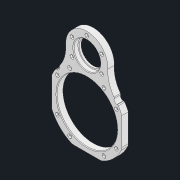
# Autodesk Inventor part: base5
Saved by Autodesk Inventor 2022 (Build 260153000, 153)
## iProperties
Created: 2021-09-16
Part Number: base5
Material: ABS プラスチック
Document SubType Name: Modeling
Designer: Yuta Kage
Density: 1.06 g/cm^3
Appearance: 滑らか - 白
Author: Yuta Kage
Autodesk Inventor part; units mm, degrees
ref_plane "YZ Plane" through (0, 0, 0) normal (1, 0, 0) x (0, 1, 0)
ref_plane "XZ Plane" through (0, 0, 0) normal (0, 1, 0) x (-1, 0, 0)
ref_plane "XY Plane" through (0, 0, 0) normal (0, 0, 1) x (1, 0, 0)
sketch "スケッチ1" plane through (0, 0, 0) normal (0, 0, 1) x (1, 0, 0)
  circle A0 centre (0, 0) radius 47.5 construction
  circle A1 centre (0, 76.8) radius 21 construction
  circle A2 centre (0, 0) radius 59.5
  circle A3 centre (0, 76.8) radius 33
  line L0 (-55.8457, 20.5306) -> (-30.9733, 88.1867)
  line L1 (30.9733, 88.1867) -> (55.8457, 20.5306)
  line L2 (-55, 131.8) -> (55, 131.8)
  line L3 (55, 131.8) -> (55, -55)
  line L4 (55, -55) -> (-55, -55)
  line L5 (-55, -55) -> (-55, 131.8)
  line L6 (-55, 131.8) -> (55, -55) construction
  line L7 (55, 131.8) -> (-55, -55) construction
  line L8 (0, 76.8) -> (-55, 131.8)
  point P0 (0, 38.4)
  point P1 (0, 38.4)
  point P2 (55, 22.8311)
  point P3 (-55, 22.8311)
  point P4 (-55, -22.6991)
  point P5 (-22.6991, -55)
  point P6 (22.6991, -55)
  point P7 (55, -22.6991)
  point P8 (-55, 22.6991)
  point P9 (55, 22.6991)
  point P10 (24.1948, 54.3587)
  point P11 (-24.1948, 54.3587)
  dimension "d0" = 95
  dimension "d1" = 42
  dimension "d2" = 76.8
  dimension "d3" = 12
  dimension "d4" = 12
  dimension "d65" = 110
  dimension "d66" = 38.4
  dimension "d68" = 45
  constraints: 18 end point, 4 centre point, 4 point on circle, 4 tangent, 3 midpoint, 2 parallel, 2 vertical alignment, 1 coincident, 1 horizontal, 1 perpendicular
  measures "d0" diameter of A0
  measures "d1" diameter of A1
  measures "d2" distance of point (0, 0) L8.start
  measures "d3" radial gap between concentric circles of A0 A2
  measures "d4" radial gap between concentric circles of A1 A3
  measures "d65" distance of L3.end L4.end
  measures "d66" distance of point (0, 0) point (0, 38.4)
  measures "d68" angle of L2 L8
extrude "押し出し1" add sketch "スケッチ1" along normal blind 10 contours A2 L4 L5 A3 L3 | A3 A2 | A2 A3
sketch "スケッチ2" plane through (0, 0, 10) normal (0, 0, 1) x (1, 0, 0)
  circle A0 centre (0, 0) radius 47.5
  dimension "d7" = 95
  constraints: 1 centre point, 1 coincident
  measures "d7" diameter of A0
extrude "押し出し2" cut sketch "スケッチ2" against normal blind 10
chamfer "面取り1" distance 1 angle 45 1 edges at (-47.5, 0, 10)
sketch "スケッチ3" plane through (0, 0, 10) normal (0, 0, 1) x (1, 0, 0)
  arc A0 (24.1948, 54.3587) -> (-24.1948, 54.3587) centre (0, 76.8) ccw projected
  circle A1 centre (0, 76.8) radius 21
  point P0 (0, 0)
  point P1 (31.1369, 90.9313)
  point P2 (-31.1369, 90.9313)
  dimension "d13" = 42
  constraints: 1 centre point, 1 coincident
  measures "d13" diameter of A1
extrude "押し出し3" cut sketch "スケッチ3" against normal blind 7
chamfer "面取り2" distance 1 angle 45 1 edges at (-21, 76.8, 10)
sketch "スケッチ4" plane through (0, 76.8, 3) normal (0, 0, 1) x (1, 0, 0)
  circle A0 centre (0, 0) radius 21 projected
  circle A1 centre (0, 0) radius 19
  point P0 (0, -76.8)
  dimension "d19" = 2
  constraints: 1 centre point
  measures "d19" radial gap between concentric circles of A0 A1
extrude "押し出し4" cut sketch "スケッチ4" against normal through all contours A1
sketch "スケッチ5" plane through (0, 0, 0) normal (0, 0, -1) x (-1, 0, 0)
  arc A0 (-55, -22.6991) -> (-22.6991, -55) centre (0, 0) ccw projected
  arc A1 (-50.4796, 17.7219) -> (50.4796, 17.7219) centre (0, 0) ccw
  circle A2 centre (0, 0) radius 47.5 projected
  arc A3 (24.1948, 54.3587) -> (-24.1948, 54.3587) centre (0, 76.8) ccw projected
  arc A4 (55, 22.6991) -> (24.1948, 54.3587) centre (0, 0) ccw projected
  arc A5 (25.4757, 85.7437) -> (-25.4757, 85.7438) centre (0, 76.8) ccw
  line L0 (25.4757, 85.7437) -> (50.4796, 17.7219)
  arc A6 (-50.4796, 17.7219) -> (50.4796, 17.7219) centre (0, 0) ccw
  line L1 (-50.4796, 17.7219) -> (-25.4757, 85.7438)
  line L2 (-55, -22.6991) -> (-55, 22.6991) projected
  line L3 (22.6991, -55) -> (-22.6991, -55) projected
  arc A7 (22.6991, -55) -> (55, -22.6991) centre (0, 0) ccw projected
  line L4 (55, 22.6991) -> (55, -22.6991) projected
  arc A8 (-24.1948, 54.3587) -> (-55, 22.6991) centre (0, 0) ccw projected
  arc A9 (-55, -22.6991) -> (-22.6991, -55) centre (0, 0) ccw projected
  point P0 (56.1408, 19.7094)
  point P1 (-56.1408, 19.7094)
  point P2 (-46.3324, -26.75)
  point P3 (-26.75, -46.3324)
  point P4 (0, -53.5)
  point P5 (26.75, -46.3324)
  point P6 (46.3324, -26.75)
  point P7 (53.5, 0)
  point P8 (46.3324, 26.75)
  point P9 (26.75, 46.3324)
  point P10 (-23.3827, 90.3)
  point P11 (-23.3827, 63.3)
  point P12 (0, 49.8)
  point P13 (23.3827, 63.3)
  point P14 (0, 53.5)
  point P15 (-26.75, 46.3324)
  point P16 (-46.3324, 26.75)
  point P17 (-53.5, 0)
  point P18 (23.3827, 90.3)
  point P19 (0, 103.8)
  dimension "d25" = 360
  dimension "d53" = 6
  dimension "d56" = 360
  dimension "d64" = 0
  constraints: 9 point on circle, 4 end point, 3 centre point, 20 other
  measures "d53" radial gap between concentric circles of A3 A5
  measures "d64" horizontal distance of point (0, 53.5) point (0, -53.5)
hole "穴1" at (0, 103.8, 0) at (-23.3827, 90.3, 0) at (23.3827, 90.3, 0) at (23.3827, 63.3, 0) at (26.75, -46.3324, 0) at (46.3324, -26.75, 0) at (46.3324, 26.75, 0) at (26.75, 46.3324, 0) at (-26.75, 46.3324, 0) at (-46.3324, 26.75, 0) at (-23.3827, 63.3, 0) at (-46.3324, -26.75, 0) at (-26.75, -46.3324, 0) direction (0, 0, 1) diameter 3.2 end through all clearance for "Socket Head Cap Screw" size "M3" standard "Ansi Metric M Profile"
sketch "スケッチ6" plane through (0, 0, 10) normal (0, 0, 1) x (1, 0, 0)
  line L0 (-3.2332, -53.5) -> (-1.6166, -50.7)
  line L1 (-1.6166, -50.7) -> (1.6166, -50.7)
  line L2 (1.6166, -50.7) -> (3.2332, -53.5)
  line L3 (3.2332, -53.5) -> (1.6166, -56.3)
  line L4 (1.6166, -56.3) -> (-1.6166, -56.3)
  line L5 (-1.6166, -56.3) -> (-3.2332, -53.5)
  circle A0 centre (0, 0) radius 47.5 projected
  circle A1 centre (0, 76.8) radius 21 projected
  circle A2 centre (0, 76.8) radius 21 projected
  line L6 (23.95, -44.7158) -> (26.75, -43.0992)
  line L7 (23.95, -47.9489) -> (23.95, -44.7158)
  line L8 (26.75, -43.0992) -> (29.55, -44.7158)
  line L9 (29.55, -44.7158) -> (29.55, -47.9489)
  line L10 (26.75, -49.5655) -> (23.95, -47.9489)
  line L11 (29.55, -47.9489) -> (26.75, -49.5655)
  line L12 (43.0992, -26.75) -> (44.7158, -23.95)
  line L13 (44.7158, -29.55) -> (43.0992, -26.75)
  line L14 (44.7158, -23.95) -> (47.9489, -23.95)
  line L15 (47.9489, -23.95) -> (49.5655, -26.75)
  line L16 (47.9489, -29.55) -> (44.7158, -29.55)
  line L17 (49.5655, -26.75) -> (47.9489, -29.55)
  line L18 (50.7, -1.6166) -> (50.7, 1.6166)
  line L19 (53.5, -3.2332) -> (50.7, -1.6166)
  line L20 (50.7, 1.6166) -> (53.5, 3.2332)
  line L21 (53.5, 3.2332) -> (56.3, 1.6166)
  line L22 (56.3, -1.6166) -> (53.5, -3.2332)
  line L23 (56.3, 1.6166) -> (56.3, -1.6166)
  line L24 (44.7158, 23.95) -> (43.0992, 26.75)
  line L25 (47.9489, 23.95) -> (44.7158, 23.95)
  line L26 (43.0992, 26.75) -> (44.7158, 29.55)
  line L27 (44.7158, 29.55) -> (47.9489, 29.55)
  line L28 (49.5655, 26.75) -> (47.9489, 23.95)
  line L29 (47.9489, 29.55) -> (49.5655, 26.75)
  line L30 (26.75, 43.0992) -> (23.95, 44.7158)
  line L31 (29.55, 44.7158) -> (26.75, 43.0992)
  line L32 (23.95, 44.7158) -> (23.95, 47.9489)
  line L33 (23.95, 47.9489) -> (26.75, 49.5655)
  line L34 (29.55, 47.9489) -> (29.55, 44.7158)
  line L35 (26.75, 49.5655) -> (29.55, 47.9489)
  line L36 (1.6166, 50.7) -> (-1.6166, 50.7)
  line L37 (3.2332, 53.5) -> (1.6166, 50.7)
  line L38 (-1.6166, 50.7) -> (-3.2332, 53.5)
  line L39 (-3.2332, 53.5) -> (-1.6166, 56.3)
  line L40 (1.6166, 56.3) -> (3.2332, 53.5)
  line L41 (-1.6166, 56.3) -> (1.6166, 56.3)
  line L42 (-23.95, 44.7158) -> (-26.75, 43.0992)
  line L43 (-23.95, 47.9489) -> (-23.95, 44.7158)
  line L44 (-26.75, 43.0992) -> (-29.55, 44.7158)
  line L45 (-29.55, 44.7158) -> (-29.55, 47.9489)
  line L46 (-26.75, 49.5655) -> (-23.95, 47.9489)
  line L47 (-29.55, 47.9489) -> (-26.75, 49.5655)
  line L48 (-24.9993, 66.1) -> (-21.7661, 66.1)
  line L49 (-21.7661, 66.1) -> (-20.1495, 63.3)
  line L50 (-20.1495, 63.3) -> (-21.7661, 60.5)
  line L51 (-21.7661, 60.5) -> (-24.9993, 60.5)
  line L52 (-24.9993, 60.5) -> (-26.6158, 63.3)
  line L53 (-26.6158, 63.3) -> (-24.9993, 66.1)
  line L54 (0, 143.02) -> (0, -89.52) projected
  line L55 (-43.0992, 26.75) -> (-44.7158, 23.95)
  line L56 (-44.7158, 29.55) -> (-43.0992, 26.75)
  line L57 (-44.7158, 23.95) -> (-47.9489, 23.95)
  line L58 (-47.9489, 23.95) -> (-49.5655, 26.75)
  line L59 (-47.9489, 29.55) -> (-44.7158, 29.55)
  line L60 (-49.5655, 26.75) -> (-47.9489, 29.55)
  line L61 (-50.7, 1.6166) -> (-50.7, -1.6166)
  line L62 (-53.5, 3.2332) -> (-50.7, 1.6166)
  line L63 (-50.7, -1.6166) -> (-53.5, -3.2332)
  line L64 (-53.5, -3.2332) -> (-56.3, -1.6166)
  line L65 (-56.3, 1.6166) -> (-53.5, 3.2332)
  line L66 (-56.3, -1.6166) -> (-56.3, 1.6166)
  line L67 (-44.7158, -23.95) -> (-43.0992, -26.75)
  line L68 (-47.9489, -23.95) -> (-44.7158, -23.95)
  line L69 (-43.0992, -26.75) -> (-44.7158, -29.55)
  line L70 (-44.7158, -29.55) -> (-47.9489, -29.55)
  line L71 (-49.5655, -26.75) -> (-47.9489, -23.95)
  line L72 (-47.9489, -29.55) -> (-49.5655, -26.75)
  line L73 (-26.75, -43.0992) -> (-23.95, -44.7158)
  line L74 (-29.55, -44.7158) -> (-26.75, -43.0992)
  line L75 (-23.95, -44.7158) -> (-23.95, -47.9489)
  line L76 (-23.95, -47.9489) -> (-26.75, -49.5655)
  line L77 (-29.55, -47.9489) -> (-29.55, -44.7158)
  line L78 (-26.75, -49.5655) -> (-29.55, -47.9489)
  line L79 (0, 0) -> (-26.75, -46.3324)
  line L80 (-1.6166, 52.6) -> (1.6166, 52.6)
  line L81 (1.6166, 52.6) -> (3.2332, 49.8)
  line L82 (-3.2332, 49.8) -> (-1.6166, 52.6)
  line L83 (3.2332, 49.8) -> (1.6166, 47)
  line L84 (1.6166, 47) -> (-1.6166, 47)
  line L85 (-1.6166, 47) -> (-3.2332, 49.8)
  line L86 (20.1495, 63.3) -> (21.7661, 66.1)
  line L87 (21.7661, 66.1) -> (24.9993, 66.1)
  line L88 (21.7661, 60.5) -> (20.1495, 63.3)
  line L89 (24.9993, 66.1) -> (26.6158, 63.3)
  line L90 (26.6158, 63.3) -> (24.9993, 60.5)
  line L91 (24.9993, 60.5) -> (21.7661, 60.5)
  line L92 (21.7661, 87.5) -> (20.1495, 90.3)
  line L93 (20.1495, 90.3) -> (21.7661, 93.1)
  line L94 (24.9993, 87.5) -> (21.7661, 87.5)
  line L95 (21.7661, 93.1) -> (24.9993, 93.1)
  line L96 (24.9993, 93.1) -> (26.6158, 90.3)
  line L97 (26.6158, 90.3) -> (24.9993, 87.5)
  circle A3 centre (-23.3827, 63.3) radius 1.6 projected
  line L98 (0, 76.8) -> (-23.3827, 63.3)
  line L99 (1.6166, 101) -> (-1.6166, 101)
  line L100 (-1.6166, 101) -> (-3.2332, 103.8)
  line L101 (3.2332, 103.8) -> (1.6166, 101)
  line L102 (-3.2332, 103.8) -> (-1.6166, 106.6)
  line L103 (-1.6166, 106.6) -> (1.6166, 106.6)
  line L104 (1.6166, 106.6) -> (3.2332, 103.8)
  line L105 (-20.1495, 90.3) -> (-21.7661, 87.5)
  line L106 (-21.7661, 87.5) -> (-24.9993, 87.5)
  line L107 (-21.7661, 93.1) -> (-20.1495, 90.3)
  line L108 (-24.9993, 87.5) -> (-26.6158, 90.3)
  line L109 (-26.6158, 90.3) -> (-24.9993, 93.1)
  line L110 (-24.9993, 93.1) -> (-21.7661, 93.1)
  point P0 (0, -53.5)
  point P1 (0, -53.5)
  point P2 (26.75, -46.3324)
  point P3 (46.3324, -26.75)
  point P4 (53.5, 0)
  point P5 (46.3324, 26.75)
  point P6 (26.75, 46.3324)
  point P7 (0, 53.5)
  point P8 (-26.75, 46.3324)
  point P9 (-46.3324, 26.75)
  point P10 (-53.5, 0)
  point P11 (-46.3324, -26.75)
  point P12 (0, 47.5)
  point P13 (0, -47.5)
  point P14 (0, 49.8)
  point P15 (0, 49.8)
  point P16 (23.3827, 63.3)
  point P17 (23.3827, 63.3)
  point P18 (23.3827, 90.3)
  point P19 (23.3827, 90.3)
  point P20 (0, 103.8)
  point P21 (0, 103.8)
  point P22 (-23.3827, 90.3)
  point P23 (-23.3827, 90.3)
  dimension "d40" = 5.6
  dimension "d43" = 360
  dimension "d59" = 5.6
  dimension "d62" = 360
  constraints: 220 end point, 5 coincident, 2 perpendicular, 268 other
  measures "d40" distance between parallel lines of L4 L1
  measures "d59" distance between parallel lines of L49 L52
extrude "押し出し5" cut sketch "スケッチ6" against normal blind 3 contours L6 L8 L9 L11 L10 L7 | L12 L14 L15 L17 L16 L13 | L24 L26 L27 L29 L28 L25 | L30 L32 L33 L35 L34 L31 | L42 L44 L45 L47 L46 L43 | L48 L49 L50 L51 L52 L53 | L103 L104 L101 L99 L54 | L54 L99 L100 L102 L103 | L55 L57 L58 L60 L59 L56 | L67 L69 L70 L72 L71 L68 | L73 L75 L76 L78 L77 L74 | L86 L87 L89 L90 L91 L88 | L92 L93 L95 L96 L97 L94 | A3 | L105 L106 L108 L109 L110 L107
fillet "フィレット1" radius 10 4 edges at (55, -22.6991, 5) (22.6991, -55, 5) (-22.6991, -55, 5) (-55, -22.6991, 5)
fillet "フィレット2" radius 50 2 edges at (24.1948, 54.3587, 5) (-24.1948, 54.3587, 5)
sketch "スケッチ7" plane through (0, 0, 0) normal (0, 0, 1) x (1, 0, 0)
  circle A0 centre (0, 76.8) radius 21 projected
  line L0 (49.05, 38.4) -> (47.15, 38.4) construction
  line L1 (49.05, 42.9) -> (47.15, 42.9)
  line L2 (47.15, 33.9) -> (49.05, 33.9)
  arc A1 (49.05, 33.9) -> (49.05, 42.9) centre (49.05, 38.4) ccw
  arc A2 (47.15, 42.9) -> (47.15, 33.9) centre (47.15, 38.4) ccw
  line L3 (47.15, 42.9) -> (60.9783, 42.9)
  line L4 (60.9783, 42.9) -> (60.9783, 33.9)
  line L5 (60.9783, 33.9) -> (47.15, 33.9)
  line L6 (47.15, 33.9) -> (47.15, 42.9)
  point P0 (0, 0)
  point P1 (48.1, 38.4)
  point P2 (49.05, 42.9)
  dimension "d72" = 76.8
  dimension "d77" = 4.5
  dimension "d78" = 38.4
  dimension "d79" = 1.9
  dimension "d82" = 48.1
  constraints: 16 end point, 4 point on circle, 4 tangent, 3 parallel, 2 centre point, 2 horizontal, 1 midpoint, 1 perpendicular
  measures "d72" distance of point (0, 0) A0.centre
  measures "d77" radius of A2
  measures "d78" distance from line of point (0, 0) L0
  measures "d79" distance of L1.start L1.end
  measures "d82" horizontal distance of point (0, 0) point (48.1, 38.4)
extrude "押し出し6" cut sketch "スケッチ7" along normal through all contours A1 L2 L6 L1 | L3 L4 L5 A1 | L6 A2
fillet "フィレット3" radius 2 2 edges at (48.8983, 33.9, 5) (43.3958, 40.8811, 5)
mirror "ミラー1" about plane through (0, 0, 0) normal (1, 0, 0) of "押し出し6", "フィレット3"
fillet_without_effect "フィレット4"
equation "\"d4\" = d3"
equation "\"d66\" = 0.5 * d2"
equation "\"d78\" = 0.5 * d72"
